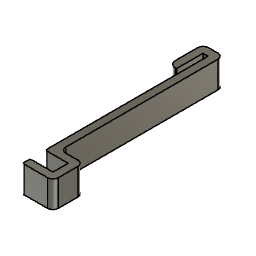
holder v1 (Autodesk Fusion 360 design; units mm, degrees)
Autodesk Fusion 360 part; units mm, degrees
sketch "Sketch1" plane through (0, 0, 0) normal (0, 0, 1) x (1, 0, 0)
  line L0 (0, 8.5) -> (0, 38)
  line L1 (8.5, 0) -> (9.5, 0)
  line L2 (10, 0.5) -> (10, 35)
  line L3 (10, 35) -> (16.6, 35)
  line L4 (16.6, 35) -> (16.6, -177.5)
  line L5 (18.6, -179.5) -> (26.6, -179.5)
  line L6 (26.6, -162.5) -> (26.6, 38)
  line L7 (19.6, 45) -> (7, 45)
  line L8 (26.6, -179.5) -> (56.6, -179.5)
  line L9 (56.6, -179.5) -> (56.6, -176.5)
  line L10 (49.6, -169.5) -> (33.6, -169.5)
  line L11 (56.6, -179.5) -> (56.6, -202.5)
  line L12 (49.6, -209.5) -> (46.6, -209.5)
  line L13 (46.6, -209.5) -> (46.6, -179.5)
  line L14 (46.6, -209.5) -> (18.6, -209.5)
  line L15 (16.6, -207.5) -> (16.6, -201.5)
  line L16 (18.6, -199.5) -> (46.6, -199.5)
  arc A0 (0, 8.5) -> (8.5, 0) centre (8.5, 8.5) ccw
  arc A1 (9.5, 0) -> (10, 0.5) centre (9.5, 0.5) ccw
  arc A2 (7, 45) -> (0, 38) centre (7, 38) ccw
  arc A3 (26.6, 38) -> (19.6, 45) centre (19.6, 38) ccw
  arc A4 (16.6, -177.5) -> (18.6, -179.5) centre (18.6, -177.5) ccw
  arc A5 (18.6, -199.5) -> (16.6, -201.5) centre (18.6, -201.5) ccw
  arc A6 (16.6, -207.5) -> (18.6, -209.5) centre (18.6, -207.5) ccw
  arc A7 (56.6, -176.5) -> (49.6, -169.5) centre (49.6, -176.5) ccw
  arc A8 (49.6, -209.5) -> (56.6, -202.5) centre (49.6, -202.5) ccw
  arc A9 (26.6, -162.5) -> (33.6, -169.5) centre (33.6, -162.5) ccw
  point P0 (0, 45)
  point P1 (10, 0)
  point P2 (16.6, -179.5)
  point P3 (56.6, -169.5)
  point P4 (56.6, -209.5)
  point P5 (16.6, -209.5)
  point P6 (16.6, -199.5)
  dimension "d1" = 45
  dimension "d2" = 10
  dimension "d3" = 35
  dimension "d4" = 6.6
  dimension "d5" = 10
  dimension "d6" = 214.5
  dimension "d7" = 30
  dimension "d8" = 10
  dimension "d9" = 30
  dimension "d10" = 10
  dimension "d11" = 30
  dimension "d12" = 10
  dimension "d13" = 8.5
  dimension "d14" = 0.5
  dimension "d15" = 7
  dimension "d16" = 7
  dimension "d17" = 2
  dimension "d18" = 2
  dimension "d19" = 2
  dimension "d20" = 7
  dimension "d21" = 7
  dimension "d22" = 7
  constraint vertical L0
  constraint perpendicular L0 L1
  constraint perpendicular L1 L2
  constraint perpendicular L2 L3
  constraint perpendicular L3 L4
  constraint perpendicular L4 L5
  constraint perpendicular L5 L6
  constraint perpendicular L0 L7
  constraint perpendicular L6 L8
  constraint perpendicular L8 L9
  constraint perpendicular L6 L10
  constraint perpendicular L8 L11
  constraint perpendicular L11 L12
  constraint coincident L8 L13.end
  constraint perpendicular L8 L13
  constraint perpendicular L13 L14
  constraint perpendicular L14 L15
  constraint coincident L13 L16.end
  constraint perpendicular L13 L16
  constraint coincident origin L0
  constraint coincident origin L1
  constraint tangent L0 A0
  constraint tangent L1 A0
  constraint coincident P1 L2
  constraint coincident P1 L1
  constraint tangent L2 A1
  constraint tangent L1 A1
  constraint coincident P0 L7
  constraint coincident P0 L0
  constraint tangent L7 A2
  constraint tangent L0 A2
  constraint tangent L7 A3
  constraint tangent L6 A3
  constraint coincident P2 L4
  constraint coincident P2 L5
  constraint tangent L4 A4
  constraint tangent L5 A4
  constraint coincident P6 L16
  constraint coincident P6 L15
  constraint tangent L16 A5
  constraint tangent L15 A5
  constraint coincident P5 L15
  constraint coincident P5 L14
  constraint tangent L15 A6
  constraint tangent L14 A6
  constraint coincident P3 L10
  constraint coincident P3 L9
  constraint tangent L10 A7
  constraint tangent L9 A7
  constraint coincident P4 L11
  constraint coincident P4 L12
  constraint tangent L11 A8
  constraint tangent L12 A8
  constraint coincident L5.end L6
  constraint tangent L6 A9
  constraint tangent L10 A9
  measures "d1" distance of origin P0
  measures "d2" distance of origin P1
  measures "d3" distance of P1 L2.end
  measures "d4" distance of L2.end L3.end
  measures "d5" distance of P2 L5.end
  measures "d6" distance of L3.end P2
  measures "d7" distance of L5.end L8.end
  measures "d8" distance of L8.end P3
  measures "d9" distance of L8.end P4
  measures "d10" distance of P4 L12.end
  measures "d11" distance of L12.end P5
  measures "d12" distance of P5 P6
  measures "d13" radius of A0
  measures "d14" radius of A1
  measures "d15" radius of A2
  measures "d16" radius of A3
  measures "d17" radius of A4
  measures "d18" radius of A5
  measures "d19" radius of A6
  measures "d20" radius of A7
  measures "d21" radius of A8
  measures "d22" radius of A9
extrude "Extrude1" add sketch "Sketch1" along normal blind 35
